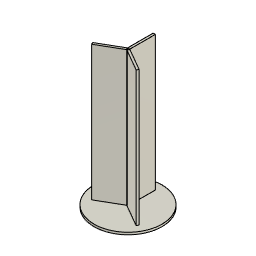
BottomLid v4 (Autodesk Fusion 360 design; units mm, degrees)
Autodesk Fusion 360 part; units mm, degrees
sketch "Sketch1" plane through (0, 0, 0) normal (0, 0, 1) x (1, 0, 0)
  circle A0 centre (0, 0) radius 31
  dimension "d1" = 62
  constraint coincident A0.centre origin
  measures "d1" diameter of A0
extrude "Extrude1" add sketch "Sketch1" along normal blind 2 makes body 1
sketch "Sketch2" plane through (0, 0, 2) normal (0, 0, 1) x (-1, 0, 0)
  circle A0 centre (0, 0) radius 31
  line L0 (-1, 0) -> (1, 0)
  line L1 (1, 0) -> (1, -24)
  line L2 (1, -24) -> (-1, -24)
  line L3 (-1, -24) -> (-1, 0)
  line L4 (21.2846, 11.134) -> (0.5, -0.866)
  line L5 (20.2846, 12.866) -> (21.2846, 11.134)
  line L6 (-0.5, 0.866) -> (20.2846, 12.866)
  line L7 (0.5, -0.866) -> (-0.5, 0.866)
  line L8 (-20.2846, 12.866) -> (0.5, 0.866)
  line L9 (-21.2846, 11.134) -> (-20.2846, 12.866)
  line L10 (-0.5, -0.866) -> (-21.2846, 11.134)
  line L11 (0.5, 0.866) -> (-0.5, -0.866)
  dimension "d7" = 360
  constraint horizontal L0
  constraint vertical L1
  constraint horizontal L2
  constraint vertical L3
extrude "Extrude2" add sketch "Sketch2" along normal blind 123 separate body contours L0 L3 L6 L7 L8 L9 L10 | L0 L1 L4 L5 L6 L8 L11 | L1 L2 L3 L4 L7 L10 L11 makes body 2 at (-6.7615, -5.0585, 43)
